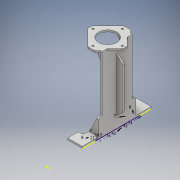
# Autodesk Inventor part: X axis screw support
Saved by Autodesk Inventor 2018 (Build 220112000, 112)
## iProperties
Created: 2017-06-27
Part Number: X axis screw support
Material: Generic
Document SubType Name: Modeling
Designer: M228544
Density: 1 g/cm^3
Appearance: Default
Author: M228544
Autodesk Inventor part; units mm, degrees
ref_plane "YZ Plane" through (0, 0, 0) normal (1, 0, 0) x (0, 1, 0)
ref_plane "XZ Plane" through (0, 0, 0) normal (0, 1, 0) x (-1, 0, 0)
ref_plane "XY Plane" through (0, 0, 0) normal (0, 0, 1) x (1, 0, 0)
sketch "Sketch1" plane through (0, 0, 0) normal (0, 0, 1) x (1, 0, 0)
  line L0 (0, 343) -> (-48.5, 343) projected
  line L1 (0, 343) -> (0, 113)
  line L2 (0, 113) -> (-48.5, 113)
  line L3 (-48.5, 113) -> (-48.5, 148)
  line L4 (-48.5, 148) -> (-32.5, 148)
  line L5 (-32.5, 148) -> (-32.5, 203)
  line L6 (-32.5, 203) -> (-13, 203)
  line L7 (-13, 203) -> (-13, 258)
  line L8 (-13, 258) -> (-32.5, 258)
  line L9 (-32.5, 258) -> (-32.5, 313)
  line L10 (-32.5, 313) -> (-48.5, 313)
  line L11 (-48.5, 313) -> (-48.5, 343)
  point P0 (0, 0)
  dimension "d0" = 230
  dimension "d1" = 13
  dimension "d2" = 30
  dimension "d3" = 55
  dimension "d4" = 55
  dimension "d5" = 55
  dimension "d6" = 16
  constraints: 22 end point, 7 perpendicular, 3 point on line, 2 vertical, 1 horizontal
  measures "d0" distance of L0.start L1.end
  measures "d1" distance between parallel lines of L1 L7
  measures "d2" distance of L10.end L0.end
  measures "d3" distance of L8.end L9.end
  measures "d4" distance of L4.end L5.end
  measures "d5" distance of L6.end L7.end
  measures "d6" distance of L3.end L4.end
extrude "Extrusion1" add sketch "Sketch1" along normal blind 6
fillet "Fillet1" radius 7 7 edges at (-32.5, 148, 3) (-32.5, 203, 3) (-13, 203, 3) (-13, 258, 3) (-32.5, 258, 3) (-32.5, 313, 3) (-48.5, 313, 3)
sketch "Sketch2" plane through (0, 0, 6) normal (0, 0, 1) x (1, 0, 0)
  line L0 (0, 113) -> (0, 343) projected
  line L1 (-6, 180) -> (0, 180)
  line L2 (0, 180) -> (0, 280)
  line L3 (0, 280) -> (-6, 280)
  line L4 (-6, 280) -> (-6, 180)
  line L5 (-15.5, 205) -> (-48.5, 205) construction
  line L6 (-48.5, 255) -> (-15.5, 255) construction
  line L7 (-15.5, 255) -> (-15.5, 205) construction
  line L8 (-15.5, 230) -> (0, 230) construction
  point P0 (0, 0)
  dimension "d10" = 100
  dimension "d11" = 6
  constraints: 12 end point, 3 perpendicular, 2 midpoint, 2 parallel, 1 horizontal, 1 point on line
  measures "d10" distance of L1.end L2.end
  measures "d11" distance of L2.end L3.end
extrude "Extrusion2" add sketch "Sketch2" along normal blind 241
sketch "Sketch3" plane through (-6, 180, 6) normal (-1, 0, 0) x (0, 0, 1)
  line L0 (241, 0) -> (241, 100) projected
  line L1 (235, 0) -> (235, 100)
  line L2 (241, 100) -> (241, 0)
  line L3 (241, 100) -> (241, 0) projected
  line L4 (241, 0) -> (241, -10)
  line L5 (241, -10) -> (235, -10)
  line L6 (235, -10) -> (235, 0)
  line L7 (235, 100) -> (235, 110)
  line L8 (235, 110) -> (241, 110)
  line L9 (0, 100) -> (241, 100) construction
  line L10 (241, 110) -> (241, 100)
  point P0 (-6, -180)
  dimension "d14" = 6
  dimension "d17" = 10
  dimension "d18" = 10
  constraints: 16 end point, 4 perpendicular, 2 point on line, 1 parallel, 1 vertical
  measures "d14" distance of L1.end L2.start
  measures "d17" distance of L8.end L0.end
  measures "d18" distance of L0.start L4.end
extrude "Extrusion3" add sketch "Sketch3" along normal blind 85
sketch "Sketch4" plane through (0, 0, 247) normal (0, 0, 1) x (1, 0, 0)
  line L0 (-37.6569, 174.8457) -> (-87.1543, 224.3431) construction
  line L1 (-87.1543, 235.6569) -> (-37.6569, 285.1543) construction
  line L2 (-40.4853, 172.0172) -> (-89.9828, 221.5147)
  line L3 (-91, 237.468) -> (-40.4853, 287.9828)
  line L4 (-89.9828, 221.5147) -> (-91, 222.532)
  line L5 (-91, 170) -> (-91, 290) projected
  line L6 (-89.9828, 238.4853) -> (-91, 237.468)
  line L7 (-40.4853, 287.9828) -> (-38.468, 290)
  line L8 (-6, 290) -> (-91, 290) projected
  line L9 (-40.4853, 172.0172) -> (-38.468, 170)
  line L10 (-6, 170) -> (-91, 170) projected
  line L11 (-38.468, 170) -> (-91, 170)
  line L12 (-6, 170) -> (-91, 170) projected
  line L13 (-91, 170) -> (-91, 222.532)
  line L14 (-91, 237.468) -> (-91, 290)
  line L15 (23.1543, 224.3431) -> (-26.3431, 174.8457) construction
  line L16 (-26.3431, 285.1543) -> (23.1543, 235.6569) construction
  line L17 (-18.7487, 292.7487) -> (30.7487, 243.2513) construction
  line L18 (30.7487, 216.7487) -> (-18.7487, 167.2513) construction
  line L19 (-6, 180) -> (0, 180) projected
  line L20 (-6, 170) -> (-6, 180) projected
  line L21 (-6, 180) -> (-6, 170)
  line L22 (-6, 170) -> (-16, 170)
  line L23 (-6, 180) -> (-16, 170)
  line L24 (-6, 280) -> (-6, 290) projected
  line L25 (-6, 280) -> (-6, 290)
  line L26 (-6, 290) -> (-16, 290)
  line L27 (-6, 280) -> (-16, 290)
  line L28 (-38.468, 290) -> (-91, 290)
  point P0 (0, 0)
  dimension "d19" = 4
  dimension "d20" = 4
  constraints: 36 end point, 9 point on line, 6 collinear, 4 parallel, 1 perpendicular
  measures "d19" distance between parallel lines of L2 L0
  measures "d20" distance between parallel lines of L3 L1
extrude "Extrusion4" cut sketch "Sketch4" against normal blind 7
sketch "Sketch5" plane through (0, 113, 0) normal (1, 0, 0) x (0, 0, -1)
  line L0 (-241, 97) -> (-247, 97)
  line L1 (-247, 97) -> (-247, 137)
  line L2 (-247, 137) -> (-241, 137)
  line L3 (-241, 137) -> (-241, 97)
  line L4 (-247, 67) -> (-247, 167) projected
  point P0 (0, -113)
  point P1 (-247, 117)
  dimension "d25" = 6
  dimension "d26" = 40
  constraints: 8 end point, 2 midpoint, 2 parallel, 1 horizontal, 1 perpendicular
  measures "d25" distance of L1.end L2.end
  measures "d26" distance of L2.end L0.start
extrude "Extrusion5" add sketch "Sketch5" along normal blind 26
chamfer "Chamfer1" distance 13 angle 45 4 edges at (0, 210, 244) (26, 210, 244) (26, 250, 244) (0, 250, 244)
fillet "Fillet2" radius 7 10 edges at (-16, 170, 244) (0, 197.0001, 244) (26, 222.9999, 244) (26, 237.0001, 244) (0, 262.9999, 244) (-16, 290, 244) (-38.468, 290, 244) (-91, 237.468, 244) (-91, 222.532, 244) (-38.468, 170, 244)
sketch "Sketch6" plane through (0, 0, 247) normal (0, 0, 1) x (1, 0, 0)
  circle A0 centre (-32, 180.7854) radius 3.25 projected
  circle A1 centre (-81.2146, 230) radius 3.25 projected
  circle A2 centre (-32, 279.2146) radius 3.25 projected
  circle A3 centre (17.2146, 230) radius 3.25 projected
  circle A4 centre (-32, 230) radius 30 construction
  circle A5 centre (-32, 230) radius 30.5
  point P0 (0, 0)
  dimension "d33" = 0.5
  constraints: 1 centre point
  measures "d33" radial gap between concentric circles of A4 A5
extrude "Extrusion6" cut sketch "Sketch6" against normal blind 7
ref_plane "Work Plane1" through (-6, 230, 6) normal (0, -1, 0) x (1, 0, 0)
ref_plane "Work Plane2" through (-6, 190, 6) normal (0, -1, 0) x (1, 0, 0)
sketch "Sketch8" plane through (-6, 230, 6) normal (0, -1, 0) x (1, 0, 0)
  point P0 (6, -6)
sketch "Sketch9" plane through (-6, 190, 6) normal (0, -1, 0) x (1, 0, 0)
  line L0 (0, 0) -> (-25, 0)
  line L1 (0, 0) -> (0, 50)
  line L2 (0, 50) -> (-25, 0)
  point P0 (6, -6)
  dimension "d39" = 25
  dimension "d40" = 50
  constraints: 6 end point, 1 horizontal, 1 vertical
  measures "d39" distance of L0.start L0.end
  measures "d40" distance of L0.start L1.end
extrude "Extrusion8" add sketch "Sketch9" along normal blind 6
mirror "Mirror1" about plane through (-6, 230, 6) normal (0, -1, 0) of "Extrusion8"
sketch "Sketch10" plane through (-6, 190, 6) normal (0, -1, 0) x (1, 0, 0)
  line L0 (0, 235) -> (-30, 235)
  line L1 (-12.8995, 235) -> (-29.5685, 235) projected
  line L2 (0, 235) -> (0, 185)
  line L3 (0, 185) -> (-30, 235)
  point P0 (6, -6)
  dimension "d43" = 30
  dimension "d45" = 50
  constraints: 6 end point, 1 point on line, 1 vertical
  measures "d43" distance of L0.start L0.end
  measures "d45" distance of L0.start L2.end
extrude "Extrusion9" add sketch "Sketch10" against normal blind 6
mirror "Mirror2" about plane through (-6, 230, 6) normal (0, -1, 0) of "Extrusion9"
sketch "Sketch11" plane through (-6, 230, 6) normal (0, -1, 0) x (1, 0, 0)
  point P0 (6, -6)
sketch "Sketch12" plane through (-6, 230, 6) normal (0, -1, 0) x (1, 0, 0)
  line L0 (6, -6) -> (6, 235) construction
  line L1 (6, 0) -> (6, 241) projected
  line L2 (6, 120.5) -> (6, 210.5)
  line L3 (6, 120.5) -> (9.7598, 120.5) construction
  line L4 (6, 120.5) -> (6, 30.5)
  line L5 (6, 120.5) -> (96, 120.5) construction
  line L6 (6, 210.5) -> (26, 190.5)
  line L7 (6, 210.5) -> (34.2843, 210.5) construction
  line L8 (26, 190.5) -> (26, 120.5)
  line L9 (6, 30.5) -> (26, 50.5)
  line L10 (26, 50.5) -> (26, 120.5)
  dimension "d48" = 90
  dimension "d49" = 90
  dimension "d50" = 90
  dimension "d51" = 45
  dimension "d52" = 20
  constraints: 20 end point, 3 horizontal, 2 collinear, 2 equal length, 2 point on line, 1 midpoint, 1 perpendicular, 1 symmetric about line
  measures "d48" distance of L2.start L2.end
  measures "d49" distance of L2.start L4.end
  measures "d50" angle of L4 L5
  measures "d51" angle of L6 L7
  measures "d52" distance from line of L0 L6.end
extrude "Extrusion10" add sketch "Sketch12" along normal mid plane 6
fillet "Fillet3" radius 7 2 edges at (20, 230, 196.5) (20, 230, 56.5)
sketch "Sketch13" plane through (0, 0, 0) normal (0, 0, -1) x (-1, 0, 0)
  line L0 (0, 233) -> (0, 227) projected
  line L1 (0, 230) -> (0, 188)
  line L2 (0, 188) -> (24.5, 188)
  circle A0 centre (24.5, 188) radius 3.5
  line L3 (0, 230) -> (0, 156)
  line L4 (0, 113) -> (0, 180) projected
  line L5 (0, 156) -> (21.5, 156)
  circle A1 centre (21.5, 156) radius 4
  line L6 (0, 230) -> (0, 272)
  line L7 (0, 113) -> (0, 343) projected
  line L8 (0, 230) -> (0, 304)
  line L9 (0, 304) -> (21.5, 304)
  line L10 (0, 272) -> (24.5, 272)
  circle A2 centre (24.5, 272) radius 3.5
  circle A3 centre (21.5, 304) radius 4
  point P0 (0, 0)
  dimension "d56" = 42
  dimension "d57" = 24.5
  dimension "d58" = 7
  dimension "d59" = 74
  dimension "d60" = 21.5
  dimension "d61" = 8
  dimension "d62" = 42
  dimension "d63" = 74
  dimension "d64" = 7
  dimension "d65" = 8
  constraints: 16 end point, 4 centre point, 4 coincident, 3 perpendicular, 1 collinear, 1 horizontal, 1 midpoint, 1 point on line, 3 other
  measures "d56" distance of L1.start L1.end
  measures "d57" distance of L1.end L2.end
  measures "d58" diameter of A0
  measures "d59" distance of L1.start L3.end
  measures "d60" distance of L3.end L5.end
  measures "d61" diameter of A1
  measures "d62" distance of L1.start L6.end
  measures "d63" distance of L1.start L8.end
  measures "d64" diameter of A2
  measures "d65" diameter of A3
sketch "Sketch14" plane through (-6, 180, 6) normal (0, -1, 0) x (1, 0, 0)
  line L0 (0, 0) -> (0, 50) projected
  line L1 (0, 0) -> (0, 55)
  line L2 (0, 55) -> (6, 55)
  line L3 (6, -6) -> (6, 0) projected
  line L4 (6, 55) -> (6, 0)
  line L5 (6, 0) -> (0, 0) projected
  line L6 (6, 0) -> (0, 0)
  dimension "d66" = 55
  constraints: 8 end point, 3 collinear, 1 perpendicular
  measures "d66" distance of L0.start L1.end
sketch "Sketch15" plane through (-6, 280, 6) normal (-1, 0, 0) x (0, 0, 1)
  point P0 (-6, -280)
extrude "Extrusion11" add sketch "Sketch14" along normal blind 12
sketch "Sketch16" plane through (-6, 280, 6) normal (0, 1, 0) x (1, 0, 0)
  line L0 (6, 0) -> (6, -241) projected
  line L1 (6, 0) -> (6, -55)
  line L2 (6, -55) -> (0, -55)
  line L3 (0, 0) -> (0, -235) projected
  line L4 (0, -55) -> (0, 0)
  line L5 (0, 0) -> (6, 0)
  point P0 (6, 6)
  dimension "d69" = 55
  constraints: 8 end point, 2 point on line, 1 horizontal, 1 perpendicular, 1 vertical
  measures "d69" distance of L0.start L1.end
extrude "Extrusion12" add sketch "Sketch16" along normal blind 12
fillet "Fillet4" radius 7 2 edges at (-3, 292, 61) (-3, 168, 61)
sketch "Sketch17" plane through (-6, 184, 6) normal (0, -1, 0) x (1, 0, 0)
  line L0 (0, 50) -> (-25, 0) projected
  line L1 (0, 48) -> (0, 0) projected
  line L2 (0, 48) -> (0, 55) projected
  line L3 (-42.5, 0) -> (6, 0) projected
  line L4 (-25, 0) -> (0, 0) projected
  line L5 (0, 0) -> (-25, 0)
  line L6 (-25, 0) -> (0, 50)
  line L7 (0, 0) -> (0, 48) projected
  line L8 (0, 0) -> (0, 50)
  line L9 (0, 48) -> (0, 55) projected
  point P0 (6, -6)
  constraints: 6 end point, 2 collinear
extrude "Extrusion13" add sketch "Sketch17" along normal blind 16
sketch "Sketch18" plane through (-6, 190, 6) normal (0, 1, 0) x (1, 0, 0)
  line L0 (0, -50) -> (-25, 0) projected
  line L1 (-25, 0) -> (0, -50)
  line L2 (0, -50) -> (0, 0)
  line L3 (6, 0) -> (-25, 0) projected
  line L4 (-25, 0) -> (0, 0)
  line L5 (-19.5, 0) -> (-26.5, 0) projected
  point P0 (6, 6)
  constraints: 6 end point, 2 collinear, 1 point on line, 1 vertical
extrude "Extrusion14" cut sketch "Sketch18" against normal blind 16
sketch "Sketch19" plane through (-31, 276, 6) normal (0, 1, 0) x (1, 0, 0)
  line L0 (25, 0) -> (0, 0) projected
  line L1 (25, -50) -> (0, 0) projected
  line L2 (0, 0) -> (25, -50)
  line L3 (25, 0) -> (25, -48) projected
  line L4 (25, -50) -> (25, 0)
  line L5 (25, 0) -> (0, 0)
  point P0 (31, 6)
  constraints: 6 end point, 2 collinear, 1 perpendicular
extrude "Extrusion15" add sketch "Sketch19" along normal blind 16
sketch "Sketch20" plane through (-31, 270, 6) normal (0, -1, 0) x (1, 0, 0)
  line L0 (0, 0) -> (25, 50) projected
  line L1 (0, 0) -> (25, 50)
  line L2 (25, 0) -> (0, 0) projected
  line L3 (25, 50) -> (25, 0)
  line L4 (25, 0) -> (0, 0)
  point P0 (31, -6)
  constraints: 6 end point, 2 collinear, 1 perpendicular
extrude "Extrusion16" cut sketch "Sketch20" against normal blind 16
body "Solid1"
